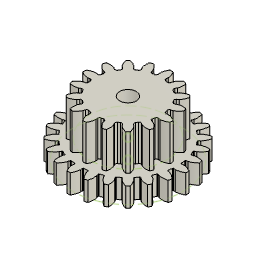
Central Gear (Autodesk Fusion 360 design; units mm, degrees)
description: Spur Gear; Module: 0.830000; Num Teeth: 24; Pressure Angle: 20.000000; Backlash: 0.00 mm
description: Spur Gear; Module: 0.880000; Num Teeth: 16; Pressure Angle: 20.000000; Backlash: 0.00 mm
Autodesk Fusion 360 part; units mm, degrees
sketch "Sketch1" plane through (0, 0, 0) normal (0, 0, 1) x (1, 0, 0) in component "Spur Gear (24 teeth)"
  circle A0 centre (0, 0) radius 8.9132
  circle A1 centre (0, 0) radius 1.5
extrude "Extrude1" add sketch "Sketch1" along normal blind 2.5 makes body 1 in component "Spur Gear (24 teeth)"
sketch "Sketch2" plane through (0, 0, 0) normal (0, 0, 1) x (1, 0, 0) in component "Spur Gear (24 teeth)"
  spline S0 degree 5 poles (9.3291, -0.7513) (9.3333, -0.7516) (9.3416, -0.7521) (9.3541, -0.7527) (9.3707, -0.7528) (9.3915, -0.7521) (9.4124, -0.7509) (9.4332, -0.7493) (9.4541, -0.7475) (9.475, -0.7455) (9.4959, -0.7435) (9.5168, -0.7412) (9.5378, -0.7387) (9.5587, -0.7359) (9.5796, -0.7328) (9.6006, -0.7295) (9.6215, -0.7259) (9.6425, -0.7222) (9.6634, -0.7182) (9.6844, -0.7141) (9.7053, -0.7099) (9.7263, -0.7055) (9.7472, -0.7009) (9.7682, -0.6962) (9.7892, -0.6912) (9.8101, -0.6861) (9.8311, -0.6809) (9.852, -0.6754) (9.8729, -0.6699) (9.8939, -0.6642) (9.9148, -0.6583) (9.9358, -0.6523) (9.9567, -0.6461) (9.9776, -0.6399) (9.9985, -0.6334) (10.0194, -0.6268) (10.0403, -0.6201) (10.0612, -0.6133) (10.0821, -0.6063) (10.103, -0.5992) (10.1239, -0.5919) (10.1448, -0.5846) (10.1656, -0.5771) (10.1865, -0.5694) (10.2073, -0.5617) (10.2281, -0.5538) (10.249, -0.5458) (10.2698, -0.5377) (10.2906, -0.5294) (10.3114, -0.5211) (10.3321, -0.5126) (10.3529, -0.5039) (10.3737, -0.4952) (10.3944, -0.4864) (10.4151, -0.4774) (10.4359, -0.4683) (10.4566, -0.4591) (10.4773, -0.4498) (10.4979, -0.4404) (10.5186, -0.4309) (10.5393, -0.4212) (10.5599, -0.4115) (10.5805, -0.4016) (10.6011, -0.3916) (10.6217, -0.3815) (10.6423, -0.3713) (10.6629, -0.361) (10.6834, -0.3506) (10.704, -0.3401) (10.7245, -0.3295) (10.745, -0.3187) (10.7614, -0.3101) (10.7736, -0.3035) (10.7818, -0.2991) (10.7859, -0.2969) knots 0 0 0 0 0 0 0.01428571 0.02857143 0.04285714 0.05714286 0.07142857 0.08571429 0.1 0.11428571 0.12857143 0.14285714 0.15714286 0.17142857 0.18571429 0.2 0.21428571 0.22857143 0.24285714 0.25714286 0.27142857 0.28571429 0.3 0.31428571 0.32857143 0.34285714 0.35714286 0.37142857 0.38571429 0.4 0.41428571 0.42857143 0.44285714 0.45714286 0.47142857 0.48571429 0.5 0.51428571 0.52857143 0.54285714 0.55714286 0.57142857 0.58571429 0.6 0.61428571 0.62857143 0.64285714 0.65714286 0.67142857 0.68571429 0.7 0.71428571 0.72857143 0.74285714 0.75714286 0.77142857 0.78571429 0.8 0.81428571 0.82857143 0.84285714 0.85714286 0.87142857 0.88571429 0.9 0.91428571 0.92857143 0.94285714 0.95714286 0.97142857 0.98571429 1 1 1 1 1 1
  spline S1 degree 5 poles (9.3291, 0.7513) (9.3333, 0.7516) (9.3416, 0.7521) (9.3541, 0.7527) (9.3707, 0.7528) (9.3915, 0.7521) (9.4124, 0.7509) (9.4332, 0.7493) (9.4541, 0.7475) (9.475, 0.7455) (9.4959, 0.7435) (9.5168, 0.7412) (9.5378, 0.7387) (9.5587, 0.7359) (9.5796, 0.7328) (9.6006, 0.7295) (9.6215, 0.7259) (9.6425, 0.7222) (9.6634, 0.7182) (9.6844, 0.7141) (9.7053, 0.7099) (9.7263, 0.7055) (9.7472, 0.7009) (9.7682, 0.6962) (9.7892, 0.6912) (9.8101, 0.6861) (9.8311, 0.6809) (9.852, 0.6754) (9.8729, 0.6699) (9.8939, 0.6642) (9.9148, 0.6583) (9.9358, 0.6523) (9.9567, 0.6461) (9.9776, 0.6399) (9.9985, 0.6334) (10.0194, 0.6268) (10.0403, 0.6201) (10.0612, 0.6133) (10.0821, 0.6063) (10.103, 0.5992) (10.1239, 0.5919) (10.1448, 0.5846) (10.1656, 0.5771) (10.1865, 0.5694) (10.2073, 0.5617) (10.2281, 0.5538) (10.249, 0.5458) (10.2698, 0.5377) (10.2906, 0.5294) (10.3114, 0.5211) (10.3321, 0.5126) (10.3529, 0.5039) (10.3737, 0.4952) (10.3944, 0.4864) (10.4151, 0.4774) (10.4359, 0.4683) (10.4566, 0.4591) (10.4773, 0.4498) (10.4979, 0.4404) (10.5186, 0.4309) (10.5393, 0.4212) (10.5599, 0.4115) (10.5805, 0.4016) (10.6011, 0.3916) (10.6217, 0.3815) (10.6423, 0.3713) (10.6629, 0.361) (10.6834, 0.3506) (10.704, 0.3401) (10.7245, 0.3295) (10.745, 0.3187) (10.7614, 0.3101) (10.7736, 0.3035) (10.7818, 0.2991) (10.7859, 0.2969) knots 0 0 0 0 0 0 0.01428571 0.02857143 0.04285714 0.05714286 0.07142857 0.08571429 0.1 0.11428571 0.12857143 0.14285714 0.15714286 0.17142857 0.18571429 0.2 0.21428571 0.22857143 0.24285714 0.25714286 0.27142857 0.28571429 0.3 0.31428571 0.32857143 0.34285714 0.35714286 0.37142857 0.38571429 0.4 0.41428571 0.42857143 0.44285714 0.45714286 0.47142857 0.48571429 0.5 0.51428571 0.52857143 0.54285714 0.55714286 0.57142857 0.58571429 0.6 0.61428571 0.62857143 0.64285714 0.65714286 0.67142857 0.68571429 0.7 0.71428571 0.72857143 0.74285714 0.75714286 0.77142857 0.78571429 0.8 0.81428571 0.82857143 0.84285714 0.85714286 0.87142857 0.88571429 0.9 0.91428571 0.92857143 0.94285714 0.95714286 0.97142857 0.98571429 1 1 1 1 1 1
  arc A0 (10.7859, -0.2969) -> (10.7859, 0.2969) centre (0, 0) ccw
  line L0 (8.8745, -0.7154) -> (9.3291, -0.7513)
  line L1 (8.8745, 0.7154) -> (9.3291, 0.7513)
  line L2 (8.8745, -0.7154) -> (8.8745, 0.7154)
  point P0 (9.4318, -0.7494)
  point P1 (9.5351, -0.7389)
  point P2 (9.6388, -0.7228)
  point P3 (9.7429, -0.7019)
  point P4 (9.8471, -0.6767)
  point P5 (9.9514, -0.6477)
  point P6 (10.0559, -0.615)
  point P7 (10.1604, -0.5789)
  point P8 (10.2649, -0.5396)
  point P9 (10.3693, -0.497)
  point P10 (10.4737, -0.4514)
  point P11 (10.578, -0.4028)
  point P12 (10.682, -0.3513)
  point P13 (9.4318, 0.7494)
  point P14 (9.5351, 0.7389)
  point P15 (9.6388, 0.7228)
  point P16 (9.7429, 0.7019)
  point P17 (9.8471, 0.6767)
  point P18 (9.9514, 0.6477)
  point P19 (10.0559, 0.615)
  point P20 (10.1604, 0.5789)
  point P21 (10.2649, 0.5396)
  point P22 (10.3693, 0.497)
  point P23 (10.4737, 0.4514)
  point P24 (10.578, 0.4028)
  point P25 (10.682, 0.3513)
extrude "Extrude2" add sketch "Sketch2" along normal blind 2.5 bodies 1 in component "Spur Gear (24 teeth)"
fillet "Fillet1" radius 0.1 2 edges at (8.8844, -0.7162, 1.25) (8.8844, 0.7162, 1.25) on bodies 1 in component "Spur Gear (24 teeth)"
pattern_circular "C-Pattern1" count 24 over 360 about axis through (0, 0, 0) along (0, 0, 1) of "Extrude2", "Fillet1" in component "Spur Gear (24 teeth)"
sketch "Sketch3" plane through (0, 0, 0) normal (0, 0, 1) x (1, 0, 0) in component "Spur Gear (24 teeth)"
  circle A0 centre (0, 0) radius 9.96 construction
extrude "Extrude3" add 1 faces at (6.4173, 0, 2.5) along direction (0, 0, 1) blind 1 on bodies 1 bodies 1 in component "Spur Gear (24 teeth)"
sketch "Sketch1 (2)" plane through (0, 0, 0) normal (0, 0, 1) x (1, 0, 0) in component "Spur Gear (16 teeth) (1)"
  circle A0 centre (0, 0) radius 5.9332
  circle A1 centre (0, 0) radius 1.5
extrude "Extrude1'" add sketch "Sketch1 (2)" along normal blind 9 separate body makes body 2 in component "Spur Gear (16 teeth) (1)"
sketch "Sketch2 (2)" plane through (0, 0, 0) normal (0, 0, 1) x (1, 0, 0) in component "Spur Gear (16 teeth) (1)"
  spline S0 degree 5 poles (6.5732, -0.7465) (6.577, -0.7469) (6.5846, -0.7476) (6.5959, -0.7484) (6.6112, -0.7489) (6.6303, -0.7486) (6.6494, -0.7477) (6.6685, -0.7465) (6.6877, -0.745) (6.7069, -0.7434) (6.7261, -0.7416) (6.7454, -0.7397) (6.7646, -0.7375) (6.7839, -0.735) (6.8032, -0.7321) (6.8224, -0.7291) (6.8417, -0.7257) (6.861, -0.7222) (6.8803, -0.7185) (6.8997, -0.7146) (6.919, -0.7106) (6.9383, -0.7064) (6.9576, -0.702) (6.977, -0.6974) (6.9963, -0.6926) (7.0156, -0.6876) (7.0349, -0.6825) (7.0543, -0.6772) (7.0736, -0.6717) (7.0929, -0.6661) (7.1123, -0.6604) (7.1316, -0.6544) (7.1509, -0.6484) (7.1702, -0.6421) (7.1895, -0.6357) (7.2088, -0.6292) (7.2281, -0.6225) (7.2474, -0.6157) (7.2667, -0.6087) (7.286, -0.6016) (7.3052, -0.5943) (7.3245, -0.5869) (7.3437, -0.5793) (7.363, -0.5717) (7.3822, -0.5638) (7.4014, -0.5559) (7.4206, -0.5478) (7.4398, -0.5396) (7.459, -0.5312) (7.4782, -0.5227) (7.4973, -0.5141) (7.5165, -0.5053) (7.5356, -0.4965) (7.5547, -0.4874) (7.5738, -0.4783) (7.5929, -0.469) (7.612, -0.4597) (7.631, -0.4501) (7.6501, -0.4405) (7.6691, -0.4307) (7.6881, -0.4209) (7.7071, -0.4108) (7.726, -0.4007) (7.745, -0.3905) (7.7639, -0.3801) (7.7828, -0.3696) (7.8017, -0.359) (7.8206, -0.3483) (7.8394, -0.3374) (7.8582, -0.3265) (7.877, -0.3154) (7.8921, -0.3064) (7.9033, -0.2997) (7.9108, -0.2951) (7.9146, -0.2928) knots 0 0 0 0 0 0 0.01428571 0.02857143 0.04285714 0.05714286 0.07142857 0.08571429 0.1 0.11428571 0.12857143 0.14285714 0.15714286 0.17142857 0.18571429 0.2 0.21428571 0.22857143 0.24285714 0.25714286 0.27142857 0.28571429 0.3 0.31428571 0.32857143 0.34285714 0.35714286 0.37142857 0.38571429 0.4 0.41428571 0.42857143 0.44285714 0.45714286 0.47142857 0.48571429 0.5 0.51428571 0.52857143 0.54285714 0.55714286 0.57142857 0.58571429 0.6 0.61428571 0.62857143 0.64285714 0.65714286 0.67142857 0.68571429 0.7 0.71428571 0.72857143 0.74285714 0.75714286 0.77142857 0.78571429 0.8 0.81428571 0.82857143 0.84285714 0.85714286 0.87142857 0.88571429 0.9 0.91428571 0.92857143 0.94285714 0.95714286 0.97142857 0.98571429 1 1 1 1 1 1
  spline S1 degree 5 poles (6.5732, 0.7465) (6.577, 0.7469) (6.5846, 0.7476) (6.5959, 0.7484) (6.6112, 0.7489) (6.6303, 0.7486) (6.6494, 0.7477) (6.6685, 0.7465) (6.6877, 0.745) (6.7069, 0.7434) (6.7261, 0.7416) (6.7454, 0.7397) (6.7646, 0.7375) (6.7839, 0.735) (6.8032, 0.7321) (6.8224, 0.7291) (6.8417, 0.7257) (6.861, 0.7222) (6.8803, 0.7185) (6.8997, 0.7146) (6.919, 0.7106) (6.9383, 0.7064) (6.9576, 0.702) (6.977, 0.6974) (6.9963, 0.6926) (7.0156, 0.6876) (7.0349, 0.6825) (7.0543, 0.6772) (7.0736, 0.6717) (7.0929, 0.6661) (7.1123, 0.6604) (7.1316, 0.6544) (7.1509, 0.6484) (7.1702, 0.6421) (7.1895, 0.6357) (7.2088, 0.6292) (7.2281, 0.6225) (7.2474, 0.6157) (7.2667, 0.6087) (7.286, 0.6016) (7.3052, 0.5943) (7.3245, 0.5869) (7.3437, 0.5793) (7.363, 0.5717) (7.3822, 0.5638) (7.4014, 0.5559) (7.4206, 0.5478) (7.4398, 0.5396) (7.459, 0.5312) (7.4782, 0.5227) (7.4973, 0.5141) (7.5165, 0.5053) (7.5356, 0.4965) (7.5547, 0.4874) (7.5738, 0.4783) (7.5929, 0.469) (7.612, 0.4597) (7.631, 0.4501) (7.6501, 0.4405) (7.6691, 0.4307) (7.6881, 0.4209) (7.7071, 0.4108) (7.726, 0.4007) (7.745, 0.3905) (7.7639, 0.3801) (7.7828, 0.3696) (7.8017, 0.359) (7.8206, 0.3483) (7.8394, 0.3374) (7.8582, 0.3265) (7.877, 0.3154) (7.8921, 0.3064) (7.9033, 0.2997) (7.9108, 0.2951) (7.9146, 0.2928) knots 0 0 0 0 0 0 0.01428571 0.02857143 0.04285714 0.05714286 0.07142857 0.08571429 0.1 0.11428571 0.12857143 0.14285714 0.15714286 0.17142857 0.18571429 0.2 0.21428571 0.22857143 0.24285714 0.25714286 0.27142857 0.28571429 0.3 0.31428571 0.32857143 0.34285714 0.35714286 0.37142857 0.38571429 0.4 0.41428571 0.42857143 0.44285714 0.45714286 0.47142857 0.48571429 0.5 0.51428571 0.52857143 0.54285714 0.55714286 0.57142857 0.58571429 0.6 0.61428571 0.62857143 0.64285714 0.65714286 0.67142857 0.68571429 0.7 0.71428571 0.72857143 0.74285714 0.75714286 0.77142857 0.78571429 0.8 0.81428571 0.82857143 0.84285714 0.85714286 0.87142857 0.88571429 0.9 0.91428571 0.92857143 0.94285714 0.95714286 0.97142857 0.98571429 1 1 1 1 1 1
  arc A0 (7.9146, -0.2928) -> (7.9146, 0.2928) centre (0, 0) ccw
  line L0 (5.8854, -0.6695) -> (6.5732, -0.7465)
  line L1 (5.8854, 0.6695) -> (6.5732, 0.7465)
  line L2 (5.8854, -0.6695) -> (5.8854, 0.6695)
  point P0 (6.667, -0.7465)
  point P1 (6.7617, -0.7377)
  point P2 (6.857, -0.7229)
  point P3 (6.9527, -0.7031)
  point P4 (7.0488, -0.6787)
  point P5 (7.145, -0.6502)
  point P6 (7.2414, -0.6178)
  point P7 (7.3379, -0.5816)
  point P8 (7.4344, -0.5419)
  point P9 (7.5308, -0.4987)
  point P10 (7.6271, -0.4521)
  point P11 (7.7232, -0.4022)
  point P12 (7.819, -0.3491)
  point P13 (6.667, 0.7465)
  point P14 (6.7617, 0.7377)
  point P15 (6.857, 0.7229)
  point P16 (6.9527, 0.7031)
  point P17 (7.0488, 0.6787)
  point P18 (7.145, 0.6502)
  point P19 (7.2414, 0.6178)
  point P20 (7.3379, 0.5816)
  point P21 (7.4344, 0.5419)
  point P22 (7.5308, 0.4987)
  point P23 (7.6271, 0.4521)
  point P24 (7.7232, 0.4022)
  point P25 (7.819, 0.3491)
extrude "Extrude2'" add sketch "Sketch2 (2)" along normal blind 9 bodies 2 in component "Spur Gear (16 teeth) (1)"
fillet "Fillet1'" radius 0.3 2 edges at (5.8952, -0.6706, 4.5) (5.8952, 0.6706, 4.5) on bodies 2 in component "Spur Gear (16 teeth) (1)"
pattern_circular "C-Pattern1'" count 16 over 360 about axis through (0, 0, 0) along (0, 0, 1) of "Extrude2'", "Fillet1'" in component "Spur Gear (16 teeth) (1)"
sketch "Sketch3 (2)" plane through (0, 0, 0) normal (0, 0, 1) x (1, 0, 0) in component "Spur Gear (16 teeth) (1)"
  circle A0 centre (0, 0) radius 7.04 construction
combine "Combine1" operation add target body 2 tool bodies 1 body 1 seen with x (1, 0, 0) y (0, 1, 0) z (0, 0, 1) at (0, 0, -3.5) in component "Spur Gear (16 teeth) (1)"
extrude "Extrude3'" cut 1 faces at (4.4204, 0, 9) along direction (0, 0, -1) blind 2.5 on bodies 2 bodies 2 in component "Spur Gear (16 teeth) (1)"
component "Spur Gear (24 teeth)" placed x (1, 0, 0) y (0, 1, 0) z (0, 0, 1) at (-0.1099, -0.0291, 0.0401)
component "Spur Gear (16 teeth) (1)" placed x (1, 0, 0) y (0, 1, 0) z (0, 0, 1) at (-0.1099, -0.0291, 3.5401)
